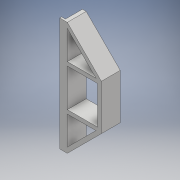
# Autodesk Inventor part: Motor_Org
Saved by Autodesk Inventor 2018 (Build 220112000, 112)
## iProperties
Created: 2018-11-07
Part Number: Motor_Org
Material: Generic
Document SubType Name: Modeling
Designer: kjy5515
Density: 1 g/cm^3
Appearance: Default
Author: kjy5515
Autodesk Inventor part; units mm, degrees
ref_plane "YZ Plane" through (0, 0, 0) normal (1, 0, 0) x (0, 1, 0)
ref_plane "XZ Plane" through (0, 0, 0) normal (0, 1, 0) x (-1, 0, 0)
ref_plane "XY Plane" through (0, 0, 0) normal (0, 0, 1) x (1, 0, 0)
sketch "Sketch1" plane through (0, 0, 0) normal (0, 1, 0) x (-1, 0, 0)
  line L0 (9, 10) -> (-7, 10)
  line L1 (-7, 10) -> (-7, -10)
  line L2 (-7, -10) -> (9, -10)
  line L3 (9, -10) -> (9, 10)
  line L4 (9, 10) -> (-7, -10) construction
  line L5 (-7, 10) -> (9, -10) construction
  line L6 (-9, 12) -> (11, 12)
  line L7 (11, 12) -> (11, -12)
  line L8 (11, -12) -> (-9, -12)
  line L9 (-9, -12) -> (-9, 12)
  line L10 (-9, 12) -> (9, 30)
  line L11 (-9, 12) -> (21.2472, 12) construction
  line L12 (11, 12) -> (11, 30)
  line L13 (-9, -12) -> (9, -30)
  line L14 (-9, -12) -> (29.5291, -12) construction
  line L15 (11, -12) -> (11, -30)
  line L16 (9, 12) -> (9, 29.1716)
  line L17 (-6.1716, -12) -> (9, -27.1716)
  line L18 (9, -27.1716) -> (9, -12)
  line L19 (11, 12) -> (11, 10)
  line L20 (11, 12) -> (9, 12)
  line L21 (-8.1716, 12) -> (-9, 12)
  line L22 (-9, -12) -> (-6.1716, -12)
  line L23 (11, -12) -> (9, -12)
  line L24 (9, 29.1716) -> (9, 30)
  line L25 (9, 30) -> (11, 30)
  line L26 (9, -27.1716) -> (11, -27.1716)
  line L27 (9, -27.1716) -> (9, -30)
  line L28 (9, -30) -> (11, -30)
  line L29 (11, 12) -> (9, 12)
  line L30 (-8.1716, 12) -> (-9, 12)
  line L31 (-6.1716, -12) -> (9, -12)
  line L32 (11, -12) -> (9, -12)
  line L33 (9, 30) -> (9, 28)
  line L34 (9, 27.1716) -> (-6.1716, 12)
  line L35 (9, 27.1716) -> (9, 30)
  line L36 (9, 27.1716) -> (-6.1716, 12)
  line L37 (-9, 12) -> (-6.1716, 12)
  line L38 (9, 30) -> (-9, 12)
  point P0 (0, 0)
  point P1 (1, 0)
  dimension "d0" = 16
  dimension "d1" = 20
  dimension "d2" = 2
  dimension "d3" = 45
  dimension "d4" = 45
  dimension "d5" = 2
  dimension "d6" = 2
  dimension "d12" = 2
  constraints: 78 end point, 9 collinear, 9 point on line, 6 parallel, 5 horizontal, 5 perpendicular, 4 vertical, 2 midpoint, 3 other
  measures "d0" distance of L2.end L1.end
  measures "d1" distance of L2.end L0.start
  measures "d2" distance between parallel lines of L0 L6
  measures "d3" angle of L11 L10
  measures "d4" angle of L13 L14
  measures "d5" distance between parallel lines of L12 L16
  measures "d6" distance between parallel lines of L13 L17
  measures "d12" distance between parallel lines of L10 L34
extrude "Extrusion2" add sketch "Sketch1" along normal blind 10 contours L10 L24 L16 L34 L6 | L6 L7 L8 L9 | L8 L17 L27 L13 | L25 L12 L6 L16 L24 | L27 L26 L15 L28 | L8 L15 L26 L18
sketch "Sketch3" plane through (0, 0, 0) normal (0, -1, 0) x (1, 0, 0)
  line L0 (-11, 30) -> (-13, 30)
  line L1 (-13, 30) -> (-13, -30)
  line L2 (-13, -30) -> (-11, -30)
  line L3 (-11, -30) -> (-11, 30) projected
  line L4 (-11, -30) -> (-11, 30)
  point P0 (0, 0)
  dimension "d15" = 2
  dimension "d16" = 60
  constraints: 8 end point, 3 perpendicular, 1 horizontal
  measures "d15" distance of L0.start L0.end
  measures "d16" distance of L0.end L1.end
extrude "Extrusion3" add sketch "Sketch3" against normal blind 1
body "Solid2"
